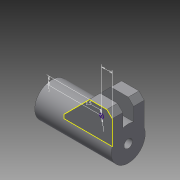
# Autodesk Inventor part: Coupler
Saved by Autodesk Inventor 2014 SP1 (Build 180222100, 222)
## iProperties
Created: 2014-01-24
Part Number: Coupler
Material: Generic
Document SubType Name: Modeling
Designer: tom
Density: 1 g/cm^3
Appearance: Default
Author: tom
Autodesk Inventor part; units mm, degrees
ref_plane "YZ Plane" through (0, 0, 0) normal (1, 0, 0) x (0, 1, 0)
ref_plane "XZ Plane" through (0, 0, 0) normal (0, 1, 0) x (-1, 0, 0)
ref_plane "XY Plane" through (0, 0, 0) normal (0, 0, 1) x (1, 0, 0)
sketch "Sketch1" plane through (0, 0, 0) normal (1, 0, 0) x (0, 1, 0)
  circle A0 centre (0, 0) radius 3.175
  circle A1 centre (0, 0) radius 6.35
  dimension "d0" = 6.35
  dimension "d1" = 12.7
  constraints: 2 centre point, 2 coincident
  measures "d0" diameter of A0
  measures "d1" diameter of A1
extrude "Extrusion1" add sketch "Sketch1" along normal blind 25.4
sketch "Sketch2" plane through (25.4, 0, 0) normal (1, 0, 0) x (0, 0, -1)
  circle A0 centre (0, 0) radius 6.35 projected
  circle A1 centre (0, 0) radius 1.5875
  circle A2 centre (0, 0) radius 6.35
  dimension "d4" = 3.175
  constraints: 2 centre point, 2 coincident, 1 concentric
  measures "d4" diameter of A1
extrude "Extrusion2" add sketch "Sketch2" along normal blind 3.175
sketch "Sketch3" plane through (28.575, 0, 0) normal (1, 0, 0) x (0, 0, -1)
  circle A0 centre (0, 0) radius 6.35
  line L0 (2, 16.026815) -> (2, 6.026815)
  line L1 (2, 16.026815) -> (6, 16.026815)
  line L2 (6, 16.026815) -> (6, 2.079062)
  line L3 (-2, 16.026815) -> (-2, 6.026815)
  line L4 (-2, 16.026815) -> (-6, 16.026815)
  line L5 (-6, 16.026815) -> (-6, 2.079062)
  dimension "d11" = 4
  dimension "d12" = 10
  dimension "d13" = 10
  constraints: 12 end point, 4 perpendicular, 4 point on circle
  measures "d11" distance of L3.start L4.end
  measures "d12" distance of L0.end L0.start
  measures "d13" distance of L3.end L3.start
extrude "Extrusion3" add sketch "Sketch3" against normal blind 18 contours A0 L0 L1 L2 | L5 L4 L3 A0
chamfer "Chamfer1" distance 9 angle 45 2 edges at (10.575, 16.0268, 4) (10.575, 16.0268, -4)
chamfer "Chamfer2" distance 2 angle 45 2 edges at (28.575, 16.0268, 4) (28.575, 16.0268, -4)
sketch "Sketch5" plane through (10.575, 2.079062, 6) normal (0, 0, 1) x (1, 0, 0)
  line L0 (16, 13.947753) -> (9, 13.947753)
  line L1 (18, 11.947753) -> (18, 0)
  circle A0 centre (13, 8.947753) radius 0.75
  point P0 (-10.575, -2.079062)
  dimension "d30" = 1.5
  dimension "d31" = 5
  dimension "d32" = 5
  constraints: 1 centre point
  measures "d30" diameter of A0
  measures "d31" distance from line of L0 A0.centre
  measures "d32" distance from line of A0.centre L1
extrude "Extrusion5" cut sketch "Sketch5" against normal blind 15
sketch "Sketch6" plane through (28.575, 0, 0) normal (1, 0, 0) x (0, 0, -1)
  arc A0 (2, 6.026815) -> (-2, 6.026815) centre (0, 0) ccw
  line L0 (-6, 14.026815) -> (-6, 2.079062)
  line L1 (2, 6.026815) -> (-2, 6.026815)
  point P0 (-6, 3.464102)
  constraints: 2 end point, 1 perpendicular, 1 point on circle
extrude "Extrusion6" cut sketch "Sketch6" against normal blind 6
pattern_circular "Circular Pattern3" count 3 over 360 about axis through (25.4, 0, 0) along (1, 0, 0) of "Extrusion3", "Chamfer2", "Extrusion5", "Extrusion6", "Chamfer1"
sketch "Sketch7" plane through (28.575, 0, 0) normal (1, 0, 0) x (0, 0, -1)
  line L0 (15.147578, -1.817255) -> (6, 3.464102)
  line L1 (-6, 14.026815) -> (-6, 3.464102)
  line L2 (-9.147578, -12.20956) -> (0, -6.928203)
  line L3 (-12.05829, -0.033654) -> (-6, 3.464102)
  arc A0 (-12.05829, -0.033654) -> (-11.53923, 2.065064) centre (-12.80829, 1.265384) ccw
  arc A1 (-7.558013, 8.960735) -> (-11.53923, 2.065064) centre (-7.732051, 4.464102) ccw
  arc A2 (-7.558013, 8.960735) -> (-6, 10.459613) centre (-7.5, 10.459613) ccw
  line L4 (-6, 3.464102) -> (-6, 10.459613)
  circle A3 centre (-7.732051, 4.464102) radius 1.5
  line L5 (6, 3.464102) -> (12.05829, -0.033654)
  line L6 (6, 10.459613) -> (6, 3.464102)
  arc A4 (6, 10.459613) -> (7.558013, 8.960735) centre (7.5, 10.459613) ccw
  arc A5 (11.53923, 2.065064) -> (7.558013, 8.960735) centre (7.732051, 4.464102) ccw
  arc A6 (11.53923, 2.065064) -> (12.05829, -0.033654) centre (12.80829, 1.265384) ccw
  circle A7 centre (7.732051, 4.464102) radius 1.5
  line L7 (6.05829, -10.425959) -> (0, -6.928203)
  arc A8 (6.05829, -10.425959) -> (3.981218, -11.025798) centre (5.30829, -11.724997) ccw
  arc A9 (-3.981218, -11.025798) -> (3.981218, -11.025798) centre (0, -8.928203) ccw
  arc A10 (-3.981218, -11.025798) -> (-6.05829, -10.425959) centre (-5.30829, -11.724997) ccw
  line L8 (0, -6.928203) -> (-6.05829, -10.425959)
  circle A11 centre (0, -8.928203) radius 1.5
extrude "Extrusion7" add sketch "Sketch7" against normal blind 8
body "Solid1"
